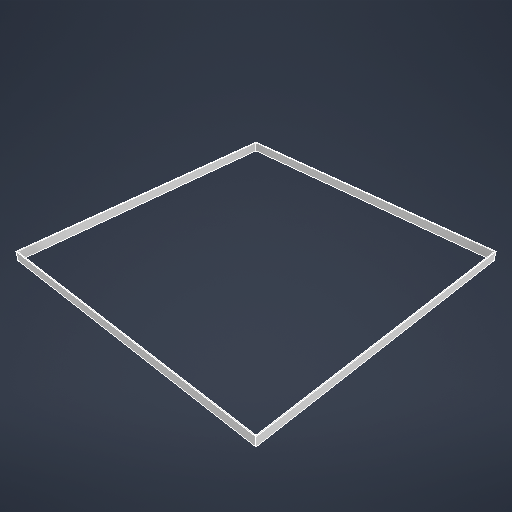
# Autodesk Inventor part: Game_Mat_Outer_Wall
Saved by Autodesk Inventor 2025 (Build 290162000, 162)
## iProperties
Created: 2024-07-08
Part Number: Game_Mat_Outer_Wall
Material: Generic
Document SubType Name: Modeling
Designer: Garfieldcmix
Density: 1 g/cm^3
Appearance: Default
Author: Garfieldcmix
Autodesk Inventor part; units mm, degrees
ref_plane "YZ Plane" through (0, 0, 0) normal (1, 0, 0) x (0, 1, 0)
ref_plane "XZ Plane" through (0, 0, 0) normal (0, 1, 0) x (-1, 0, 0)
ref_plane "XY Plane" through (0, 0, 0) normal (0, 0, 1) x (1, 0, 0)
sketch "Sketch1" plane through (0, 0, 0) normal (0, 1, 0) x (-1, 0, 0)
  line L0 (0, 0) -> (3020, 0)
  line L1 (3020, 0) -> (3020, -3020)
  line L2 (3020, -3020) -> (0, -3020)
  line L3 (0, -3020) -> (0, 0)
  line L4 (10, -10) -> (3010, -10)
  line L5 (3010, -10) -> (3010, -3010)
  line L6 (3010, -3010) -> (10, -3010)
  line L7 (10, -3010) -> (10, -10)
  line L8 (3020, -1510) -> (0, -1510) construction
  line L9 (3010, -1510) -> (10, -1510) construction
  point P0 (1510, -1510)
  dimension "d0" = 3020
  dimension "d1" = 3020
  dimension "d2" = 3000
  dimension "d3" = 3000
  constraints: 20 end point, 6 midpoint, 4 parallel, 2 horizontal, 2 perpendicular
  measures "d0" distance of L1.end L2.end
  measures "d1" distance of L0.end L1.end
  measures "d2" distance of L5.end L6.end
  measures "d3" distance of L4.end L5.end
extrude "Extrusion1" add sketch "Sketch1" along normal blind 100
body "Solid1"
